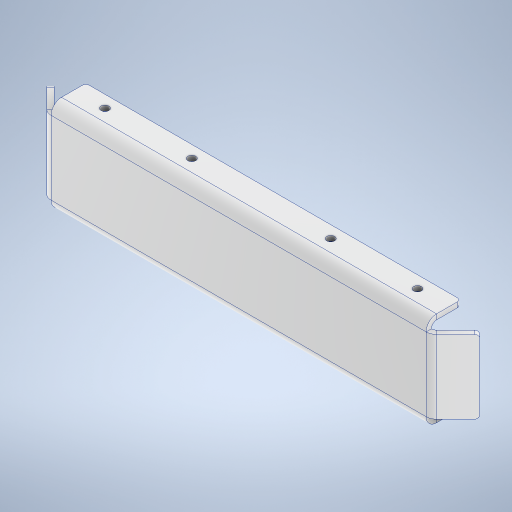
# Autodesk Inventor part: Stossfänger_04
Saved by Autodesk Inventor 2024 (Build 280153000, 153)
## iProperties
Created: 2024-03-25
Part Number: Stossfänger_04
Material: Aluminium 6061
Document SubType Name: Sheet Metal
Designer: month
Density: 2.7 g/cm^3
Sheet Metal Rule: Standard
Appearance: Aluminium - flach
Mass: 161.069 g
Surface Area: 421.44 cm^2
Volume: 59.6552 cm^3
Flat Pattern Width: 8.38717 cm
Flat Pattern Length: 25.7815 cm
Flat Pattern Area: 216.234 cm^2
Sheet Metal Width: 83,872 mm
Sheet Metal Length: 257,815 mm
Sheet Metal Area: 21623,401 mm^2
Author: month
Autodesk Inventor part; units mm, degrees
ref_plane "YZ Plane" through (0, 0, 0) normal (1, 0, 0) x (0, 1, 0)
ref_plane "XZ Plane" through (0, 0, 0) normal (0, 1, 0) x (-1, 0, 0)
ref_plane "XY Plane" through (0, 0, 0) normal (0, 0, 1) x (1, 0, 0)
sketch "Skizze1" plane through (0, 0, 0) normal (0, 1, 0) x (-1, 0, 0)
  line L0 (0, 0) -> (216, 0)
  line L1 (216, 0) -> (216, -42.3)
  line L2 (216, -42.3) -> (0, -42.3)
  line L3 (0, -42.3) -> (0, 0)
  dimension "d0" = 216
  dimension "d1" = 42.3
  constraints: 8 end point, 2 parallel, 1 horizontal, 1 perpendicular
  measures "d0" distance of L1.end L2.end
  measures "d1" distance of L2.end L0.start
extrude "Extrusion1" add sketch "Skizze1" along normal blind 3
sketch "Skizze2" plane through (0, 6, 3) normal (0, 0, 1) x (1, 0, 0)
  line L0 (-216, 0) -> (0, 0)
  line L1 (0, 0) -> (0, 14)
  line L2 (0, 14) -> (-216, 14)
  line L3 (-216, 14) -> (-216, 0)
  constraints: 6 end point, 1 horizontal, 1 perpendicular, 1 vertical
edge flange "Lasche1" height 20 angle 90 thickness 3 bend radius 3 thickness toward (0, 0, 1) relief tear relief width 3 relief depth 1.5 corner gap 3 corner form 0 edges at (-108, 3, 0) (-108, 3, -42.3) wall of the first edge with corners at (-216, 6, 3) (0, 6, 3) (0, 20, 3) (-216, 20, 3)
bend "Biegung1"
corner "Ecke1"
sketch "Skizze3" plane through (-218.1213, 3.8787, 0) normal (-0.7071068, -0.7071068, 0) x (0.7071068, -0.7071068, 0)
  line L0 (0, -42.3) -> (0, 0)
  line L1 (0, 0) -> (-17.5147, 0)
  line L2 (-17.5147, 0) -> (-17.5147, -42.3)
  line L3 (-17.5147, -42.3) -> (0, -42.3)
  constraints: 6 end point, 1 horizontal, 1 perpendicular, 1 vertical
edge flange "Lasche2" height 20 angle 45 thickness 3 bend radius 3 thickness toward (-0.7071068, -0.7071068, 0) relief tear relief width 3 relief depth 1.5 corner gap 3 corner form 0 edges at (-216, 3, -21.15) (0, 3, -21.15) wall of the first edge with corners at (-218.1213, 3.8787, -42.3) (-218.1213, 3.8787, 0) (-230.5061, 16.2635, 0) (-230.5061, 16.2635, -42.3)
bend "Biegung2"
corner "Ecke2"
sketch "Skizze4" plane through (-216, 20, 6) normal (0, 0, 1) x (1, 0, 0)
  line L0 (0, 0) -> (0, -14) projected
  line L1 (0, -7) -> (216, -7)
  line L2 (216, 0) -> (216, -14) projected
  line L3 (0, 0) -> (216, 0) projected
  line L4 (108, 0) -> (108, -14)
  line L5 (216, -14) -> (0, -14) projected
  circle A0 centre (68, -7) radius 2.25
  circle A1 centre (18, -7) radius 2.25
  circle A2 centre (148, -7) radius 2.25
  circle A3 centre (198, -7) radius 2.25
  point P0 (216, -20)
  dimension "d25" = 4.5
  dimension "d26" = 4.5
  dimension "d27" = 4.5
  dimension "d28" = 4.5
  dimension "d29" = 80
  dimension "d30" = 180
  constraints: 4 centre point, 4 end point, 4 midpoint, 4 point on line, 2 symmetric about line
  measures "d25" diameter of A0
  measures "d26" diameter of A1
  measures "d27" diameter of A2
  measures "d28" diameter of A3
  measures "d29" distance of A0.centre A2.centre
  measures "d30" distance of A3.centre A1.centre
extrude "Extrusion2" cut sketch "Skizze4" against normal blind 100 contours A1 L1 | L1 A1 | A0 L1 | L1 A0 | A2 L1 | L1 A2 | A3 L1 | L1 A3
fillet "Rundung1" radius 2 8 edges at (-231.5668, 15.2028, 0) (-231.5668, 15.2028, -42.3) (-216, 20, -46.8) (-216, 20, 4.5) (0, 20, 4.5) (15.5668, 15.2028, 0) (0, 20, -46.8) (15.5668, 15.2028, -42.3)
equation "\"d4\" = Stärke"
equation "\"d5\" = BreiteBiegungsfreistellung"
equation "\"d6\" = TiefeBiegungsfreistellung"
equation "\"d7\" = MinimalRest"
equation "\"d8\" = Übergangsradius"
equation "\"d11\" = Biegeradius"
equation "\"d12\" = GrößeEckenfreistellung"
equation "\"d13\" = Abstandsgröße"
equation "\"d14\" = JacobiRadiusGröße"
equation "\"d15\" = BreiteBiegungsfreistellung"
equation "\"d16\" = TiefeBiegungsfreistellung"
equation "\"d17\" = MinimalRest"
equation "\"d18\" = Übergangsradius"
equation "\"d21\" = Biegeradius"
equation "\"d22\" = GrößeEckenfreistellung"
equation "\"d23\" = Abstandsgröße"
equation "\"d24\" = JacobiRadiusGröße"
equation "\"Biegeradius\" = Stärke"
equation "\"BreiteBiegungsfreistellung\" = Stärke"
equation "\"TiefeBiegungsfreistellung\" = 0.5 * Stärke"
equation "\"GrößeEckenfreistellung\" = 4 * Stärke"
equation "\"MinimalRest\" = 2 * Stärke"
equation "\"Übergangsradius\" = Biegeradius"
equation "\"JacobiRadiusGröße\" = Biegeradius"
equation "\"Abstandsgröße\" = Stärke"
equation "\"Stärke\" = 3"
